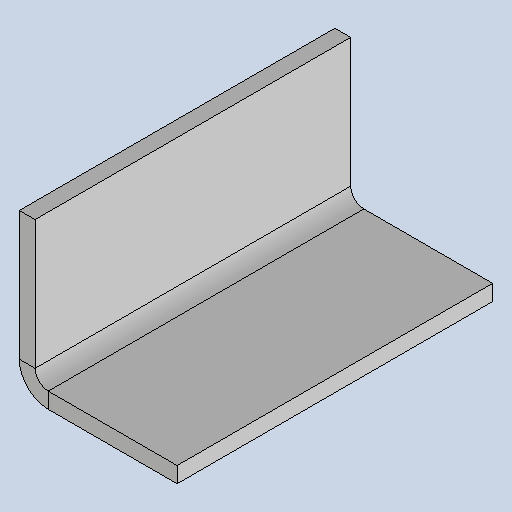
# Autodesk Inventor part: GnG frame 4.2 reinf
Saved by Autodesk Inventor 2025.3 (Build 293356030, 356C)
## iProperties
Created: 2025-10-28
Part Number: GnG frame 4.2 reinf
Material: Stainless Steel
Document SubType Name: Sheet Metal
Designer: admin
Stock Number: 1.4
Mass: 636.862 g
Surface Area: 293.027 cm^2
Volume: 79.6078 cm^3
Density: 8 g/cm^3
Flat Pattern Width: 12 cm
Flat Pattern Length: 11.0001 cm
Flat Pattern Area: 132.001 cm^2
Sheet Metal Rule: AISI304 3mm Die 32
Sheet Metal Width: 120,000 mm
Sheet Metal Length: 110,001 mm
Sheet Metal Area: 13200,106 mm^2
Appearance: Default
Author: admin
Autodesk Inventor part; units mm, degrees
ref_plane "YZ Plane" through (0, 0, 0) normal (1, 0, 0) x (0, 1, 0)
ref_plane "XZ Plane" through (0, 0, 0) normal (0, 1, 0) x (-1, 0, 0)
ref_plane "XY Plane" through (0, 0, 0) normal (0, 0, 1) x (1, 0, 0)
sketch "Sketch6" plane through (0, 0, 0) normal (0, 0, 1) x (1, 0, 0)
  line L0 (0, 0) -> (60, 0)
  line L1 (60, 0) -> (60, 120)
  line L2 (60, 120) -> (0, 120)
  line L3 (0, 120) -> (0, 0)
  dimension "d47" = 60
  dimension "d48" = 120
  measures "d47" distance of L2.end L1.end
  measures "d48" distance of L1.end L0.end
extrude "Plate3" add sketch "Sketch6" along normal blind 6
sketch "Sketch7" plane through (6, 0, 0) normal (-1, 0, 0) x (0, -1, 0)
  line L0 (-120, 0) -> (0, 0)
  line L1 (0, 0) -> (0, 60)
  line L2 (0, 60) -> (-120, 60)
  line L3 (-120, 60) -> (-120, 0)
  constraints: 6 end point, 1 horizontal, 1 perpendicular, 1 vertical
edge flange "Flange2" height 60 angle 90 thickness 6 bend radius 5 thickness toward (-1, 0, 0) relief round relief width 6 relief depth 3 edges at (0, 60, 6) wall of the first edge with corners at (6, 120, 0) (6, 0, 0) (6, 0, 60) (6, 120, 60)
bend "Bend2"
corner "Corner2"
equation "\"d46\" = Thickness"
equation "\"d49\" = BendReliefWidth"
equation "\"d50\" = BendReliefDepth"
equation "\"d51\" = MinimumRemnant"
equation "\"d52\" = TransitionRadius"
equation "\"d55\" = BendRadius"
equation "\"d56\" = CornerReliefSize"
equation "\"d57\" = GapSize"
equation "\"d58\" = JacobiRadiusSize"
equation "\"BendReliefWidth\" = Thickness"
equation "\"BendReliefDepth\" = 0.5 * Thickness"
equation "\"CornerReliefSize\" = 4 * Thickness"
equation "\"MinimumRemnant\" = 2 * Thickness"
equation "\"TransitionRadius\" = BendRadius"
equation "\"JacobiRadiusSize\" = BendRadius"
equation "\"GapSize\" = Thickness"
equation "\"Thickness\" = 6"
equation "\"BendRadius\" = 5"
body "Solid2"
